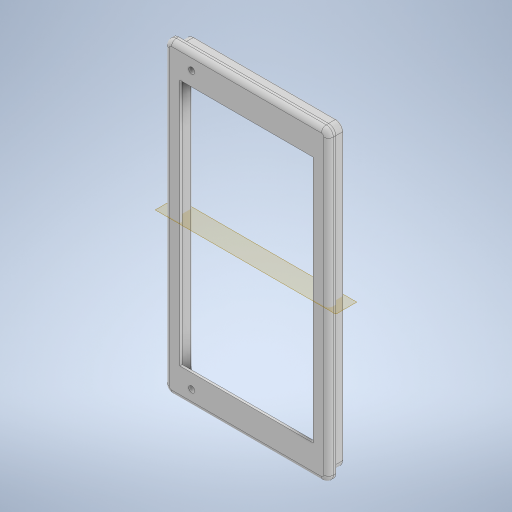
# Autodesk Inventor part: lid
Saved by Autodesk Inventor 2023 (Build 270158000, 158)
## iProperties
Created: 2022-05-07
Part Number: lid
Material: Generic
Document SubType Name: Modeling
Designer: filip
Density: 1 g/cm^3
Appearance: Default
Author: filip
Autodesk Inventor part; units mm, degrees
ref_plane "YZ Plane" through (0, 0, 0) normal (1, 0, 0) x (0, 1, 0)
ref_plane "XZ Plane" through (0, 0, 0) normal (0, 1, 0) x (-1, 0, 0)
ref_plane "XY Plane" through (0, 0, 0) normal (0, 0, 1) x (1, 0, 0)
sketch "Sketch1" plane through (0, 0, 0) normal (0, 0, 1) x (1, 0, 0)
  line L0 (34.1783, -62.3846) -> (-34.8217, -62.3846)
  line L1 (-34.8217, -62.3846) -> (-34.8217, 66.6154)
  line L2 (-34.8217, 66.6154) -> (34.1783, 66.6154)
  line L3 (34.1783, 66.6154) -> (34.1783, -62.3846)
  line L4 (34.1783, -62.3846) -> (-34.8217, 66.6154) construction
  line L5 (-34.8217, -62.3846) -> (34.1783, 66.6154) construction
  point P0 (-0.3217, 2.1154)
  dimension "d24" = 69
  dimension "d25" = 129
  constraints: 12 end point, 2 midpoint, 2 parallel, 1 horizontal, 1 perpendicular
  measures "d24" distance of L1.end L2.end
  measures "d25" distance of L0.end L1.end
extrude "Extrusion1" add sketch "Sketch1" along normal blind 3
sketch "Sketch2" plane through (0, 0, 0) normal (0, 0, -1) x (-1, 0, 0)
  line L0 (34.8217, 66.6154) -> (34.8217, -62.3846) projected
  line L1 (-34.1783, 66.6154) -> (34.8217, 66.6154) projected
  line L2 (34.8217, -62.3846) -> (-34.1783, -62.3846)
  line L3 (-34.1783, -62.3846) -> (-34.1783, 66.6154)
  line L4 (-34.1783, 66.6154) -> (34.8217, 66.6154)
  line L5 (34.8217, 66.6154) -> (34.8217, -62.3846)
  line L6 (-29.5183, -60.7246) -> (30.1617, -60.7246)
  line L7 (33.1617, -57.7246) -> (33.1617, 61.9554)
  line L8 (30.1617, 64.9554) -> (-29.5183, 64.9554)
  line L9 (-32.5183, 61.9554) -> (-32.5183, -57.7246)
  arc A0 (30.1617, -60.7246) -> (33.1617, -57.7246) centre (30.1617, -57.7246) ccw
  arc A1 (-32.5183, -57.7246) -> (-29.5183, -60.7246) centre (-29.5183, -57.7246) ccw
  arc A2 (33.1617, 61.9554) -> (30.1617, 64.9554) centre (30.1617, 61.9554) ccw
  arc A3 (-29.5183, 64.9554) -> (-32.5183, 61.9554) centre (-29.5183, 61.9554) ccw
  line L10 (-27.5183, 62.9554) -> (28.1617, 62.9554)
  line L11 (31.1617, 59.9554) -> (31.1617, -55.7246)
  line L12 (28.1617, -58.7246) -> (-27.5183, -58.7246)
  line L13 (-30.5183, -55.7246) -> (-30.5183, 59.9554)
  arc A4 (-27.5183, 62.9554) -> (-30.5183, 59.9554) centre (-27.5183, 59.9554) ccw
  arc A5 (31.1617, 59.9554) -> (28.1617, 62.9554) centre (28.1617, 59.9554) ccw
  arc A6 (28.1617, -58.7246) -> (31.1617, -55.7246) centre (28.1617, -55.7246) ccw
  arc A7 (-30.5183, -55.7246) -> (-27.5183, -58.7246) centre (-27.5183, -55.7246) ccw
  point P0 (-32.5183, 64.9554)
  dimension "d26" = 1.66
  dimension "d27" = 3
  dimension "d29" = 3
  dimension "d30" = 2
  dimension "d32" = 2
  dimension "d33" = 2
  dimension "d34" = 3
  dimension "d48" = 2
  constraints: 24 end point, 16 point on circle, 16 tangent, 8 centre point, 6 parallel, 5 equal radius, 3 perpendicular, 2 horizontal, 2 point on line, 3 other
  measures "d26" distance between parallel lines of L2 L6
  measures "d27" radius of A0
  measures "d29" radius of A3
  measures "d30" distance between parallel lines of L10 L8
  measures "d32" distance between parallel lines of L9 L13
  measures "d33" distance between parallel lines of L6 L12
  measures "d34" radius of A4
  measures "d48" distance between parallel lines of L7 L11
extrude "Extrusion2" add sketch "Sketch2" along normal blind 5 contours A1 L9 A3 L8 A2 L7 A0 L6
sketch "Sketch3" plane through (0, 0, 3) normal (0, 0, 1) x (1, 0, 0)
  line L0 (34.1783, -62.3846) -> (34.1783, 66.6154) construction
  line L1 (34.1783, 2.1154) -> (-3.6343, 2.1154) construction
  line L2 (34.1783, 66.6154) -> (-34.8217, 66.6154) construction
  line L3 (-0.3217, 66.6154) -> (-0.3217, 2.1154) construction
  line L4 (-28.3217, -49.8846) -> (27.6783, -49.8846)
  line L5 (27.6783, -49.8846) -> (27.6783, 54.1154)
  line L6 (27.6783, 54.1154) -> (-28.3217, 54.1154)
  line L7 (-28.3217, 54.1154) -> (-28.3217, -49.8846)
  line L8 (-28.3217, -49.8846) -> (27.6783, 54.1154) construction
  line L9 (27.6783, -49.8846) -> (-28.3217, 54.1154) construction
  dimension "d35" = 104
  dimension "d36" = 56
  constraints: 16 end point, 4 midpoint, 2 horizontal, 2 parallel, 2 perpendicular, 1 point on line
  measures "d35" distance of L4.end L5.end
  measures "d36" distance of L5.end L6.end
extrude "Extrusion3" cut sketch "Sketch3" against normal up to next
sketch "Sketch7" plane through (0, 0, 0) normal (0, 0, -1) x (-1, 0, 0)
  line L0 (31.1617, 62.9554) -> (-31.41, 62.9554)
  line L1 (-31.41, 62.9554) -> (-31.41, 57.6154)
  line L2 (-31.41, 57.6154) -> (31.1617, 57.6154)
  line L3 (31.1617, 57.6154) -> (31.1617, 62.9554)
  line L4 (-27.6783, 54.1154) -> (28.3217, 54.1154) projected
  line L5 (28.3217, -49.8846) -> (28.3217, 54.1154) construction
  line L6 (28.3217, 2.1154) -> (-27.6783, 2.1154) construction
  line L7 (-27.6783, -49.8846) -> (-27.6783, 54.1154) construction
  line L8 (31.1617, -58.7246) -> (-31.41, -58.7246)
  line L9 (-31.41, -58.7246) -> (-31.41, -53.3846)
  line L10 (-31.41, -53.3846) -> (31.1617, -53.3846)
  line L11 (31.1617, -53.3846) -> (31.1617, -58.7246)
  line L12 (-27.6783, -49.8846) -> (28.3217, -49.8846)
  line L13 (28.3217, 54.1154) -> (28.3217, -49.8846) construction
  line L14 (-27.6783, 54.1154) -> (-27.6783, -49.8846) construction
  line L15 (31.1617, -55.7246) -> (31.1617, 59.9554) projected
  line L16 (-27.5183, -58.7246) -> (28.1617, -58.7246) projected
  dimension "d37" = 3.5
  dimension "d51" = 0
  dimension "d52" = 0
  constraints: 24 end point, 8 symmetric about line, 2 midpoint, 2 parallel, 1 horizontal, 1 perpendicular
  measures "d37" distance between parallel lines of L4 L2
  measures "d51" distance between parallel lines of L15 L3
  measures "d52" distance between parallel lines of L16 L8
extrude "Extrusion4" add sketch "Sketch7" along normal blind 1.2
fillet "Fillet1" radius 2 4 edges at (-34.8217, 2.1154, 3) (-0.3217, 66.6154, 3) (34.1783, 2.1154, 3) (-0.3217, -62.3846, 3)
fillet "Fillet2" radius 0.5 16 edges at (-30.283, 62.0768, -5) (-31.1617, 2.1154, -5) (-30.283, -57.8459, -5) (-0.3217, -58.7246, -5) (29.6396, -57.8459, -5) (30.5183, 2.1154, -5) (29.6396, 62.0768, -5) (-0.3217, 62.9554, -5) (31.6396, 64.0768, -5) (32.5183, 2.1154, -5) (31.6396, -59.8459, -5) (-0.3217, -60.7246, -5) (-32.283, -59.8459, -5) (-33.1617, 2.1154, -5) (-32.283, 64.0768, -5) (-0.3217, 64.9554, -5)
fillet "Fillet3" radius 3 2 edges at (33.5925, 66.0297, 2.4142) (34.1783, 66.6154, 0.5)
fillet "Fillet4" radius 3 6 edges at (-34.8217, 66.6154, 0.5) (-34.2359, 66.0297, 2.4142) (-34.8217, -62.3846, 0.5) (-34.2359, -61.7988, 2.4142) (34.1783, -62.3846, 0.5) (33.5925, -61.7988, 2.4142)
sketch "Sketch10" plane through (0, 0, 3) normal (0, 0, 1) x (1, 0, 0)
  circle A0 centre (-23.3217, 60.1154) radius 1.25
  line L0 (-28.3217, 54.1154) -> (27.6783, 54.1154) projected
  line L1 (-28.3217, -49.8846) -> (-28.3217, 54.1154) projected
  point P0 (0, 0)
  dimension "d41" = 6
  dimension "d42" = 2.5
  dimension "d43" = 5
  constraints: 1 centre point
  measures "d41" distance from line of L0 A0.centre
  measures "d42" diameter of A0
  measures "d43" distance from line of L1 A0.centre
sketch "Sketch11" plane through (-28.3217, 54.1154, 3) normal (0, -1, 0) x (1, 0, 0)
  line L0 (5, 0) -> (-0.787, -8.2647)
  line L1 (0, 0) -> (56, 0) projected
  point P0 (28.3217, -3)
  dimension "d44" = 55
  constraints: 2 end point
  measures "d44" angle of L1 L0
sweep "Sweep1" cut profiles "Sketch10" path "Sketch11" path curves L0
ref_plane "Work Plane2" through (-28.3217, 2.1154, 3) normal (0, 1, 0) x (1, 0, 0)
mirror "Mirror1" about plane through (-28.3217, 2.1154, 3) normal (0, 1, 0) of "Sweep1"
sketch "Sketch12" plane through (0, 0, 0) normal (0, 0, -1) x (-1, 0, 0)
  line L0 (31.1617, -53.3846) -> (31.1617, 57.6154) projected
  line L1 (-30.5183, 57.6154) -> (-30.5183, -53.3846) projected
  line L2 (31.1617, 57.6154) -> (-30.5183, 57.6154)
  line L3 (-30.5183, 57.6154) -> (-30.5183, -53.3846)
  line L4 (-30.5183, -53.3846) -> (31.1617, -53.3846)
  line L5 (31.1617, -53.3846) -> (31.1617, 57.6154)
  point P0 (0, 0)
  point P1 (-30.5183, 57.6154)
  point P2 (31.1617, -53.3846)
  constraints: 8 end point, 2 parallel, 1 horizontal, 1 perpendicular
extrude "Extrusion5" cut sketch "Sketch12" against normal blind 2
fillet "Fillet7" radius 1.5 2 edges at (-31.1617, 2.1154, 2) (30.5183, 2.1154, 2)
fillet "Fillet7" radius 1.9 2 edges at (-0.3217, -53.3846, 2) (-0.3217, 57.6154, 2)
body "Solid1"
